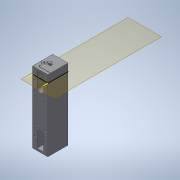
# Autodesk Inventor part: wheel-adapter-front
Saved by Autodesk Inventor 2020 (Build 240168000, 168)
## iProperties
Created: 2020-05-14
Part Number: wheel-adapter-front
Material: Ogólny
Document SubType Name: Modeling
Designer: blep
Density: 1 g/cm^3
Appearance: Domyślna
Author: blep
Autodesk Inventor part; units mm, degrees
ref_plane "YZ Plane" through (0, 0, 0) normal (1, 0, 0) x (0, 1, 0)
ref_plane "XZ Plane" through (0, 0, 0) normal (0, 1, 0) x (-1, 0, 0)
ref_plane "XY Plane" through (0, 0, 0) normal (0, 0, 1) x (1, 0, 0)
ref_plane "Płaszczyzna konstrukcyjna1" through (33, 3, -33.6408) normal (0, 1, 0) x (0, 0, 1)
sketch "Szkic1" plane through (33, 3, -33.6408) normal (0, 1, 0) x (0, 0, 1)
  line L0 (33.6408, -11) -> (70.3592, -11) projected
  line L1 (33.6408, -33) -> (33.6408, -11) projected
  line L2 (33.6408, -11) -> (70.3592, -11)
  line L3 (70.3592, -11) -> (70.3592, -33)
  line L4 (70.3592, -33) -> (33.6408, -33)
  line L5 (33.6408, -33) -> (33.6408, -11)
  constraints: 8 end point, 4 collinear, 2 parallel, 1 horizontal, 1 perpendicular
extrude "Wyciągnięcie proste1" add sketch "Szkic1" against normal blind 3
sketch "Szkic2" plane through (33, 0, -33.6408) normal (0, -1, 0) x (1, 0, 0)
  line L0 (-11, 33.6408) -> (-33, 33.6408)
  line L1 (-33, 33.6408) -> (-33, 39.6408)
  line L2 (-33, 39.6408) -> (-11, 39.6408)
  line L3 (-11, 39.6408) -> (-11, 33.6408)
  line L4 (-33, 33.6408) -> (-11, 33.6408) projected
  line L5 (-11, 33.6408) -> (-11, 70.3592) projected
  line L6 (-33, 70.3592) -> (-33, 33.6408) projected
  dimension "d2" = 6
  constraints: 8 end point, 3 collinear, 2 parallel, 1 horizontal, 1 perpendicular
  measures "d2" distance between parallel lines of L0 L2
extrude "Wyciągnięcie proste2" add sketch "Szkic2" along normal blind 20
sketch "Szkic3" plane through (22, 3, 0) normal (0, 0, -1) x (-1, 0, 0)
  circle A0 centre (18.7, -6) radius 1.25 projected
  circle A1 centre (3.3, -6) radius 1.25 projected
  circle A2 centre (3.3, -20) radius 1.25 projected
  circle A3 centre (18.7, -20) radius 1.25 projected
  circle A4 centre (11, -13) radius 2.125 projected
  circle A5 centre (18.7, -6) radius 1.5
  circle A6 centre (18.7, -20) radius 1.5
  circle A7 centre (3.3, -6) radius 1.5
  circle A8 centre (3.3, -20) radius 1.5
  point P0 (22, -3)
  dimension "d5" = 0.25
  dimension "d6" = 0.25
  dimension "d7" = 0.25
  dimension "d8" = 0.25
  constraints: 4 centre point
  measures "d5" radial gap between concentric circles of A0 A5
  measures "d6" radial gap between concentric circles of A3 A6
  measures "d7" radial gap between concentric circles of A1 A7
  measures "d8" radial gap between concentric circles of A2 A8
extrude "Wyciągnięcie proste3" cut sketch "Szkic3" against normal through all contours A0 | A1 | A2 | A3 | A4 | A5 | A6 | A7 | A8
sketch "Szkic4" plane through (33, 3, -33.6408) normal (0, 1, 0) x (1, 0, 0)
  line L0 (-33, -48.2408) -> (-22, -48.2408) construction
  line L1 (-22, -48.2408) -> (-11, -48.2408) construction
  line L2 (-11, -70.3592) -> (-11, -33.6408) projected
  line L3 (-33, -33.6408) -> (-33, -70.3592) projected
  line L4 (-11, -33.6408) -> (-33, -33.6408) projected
  line L5 (-22, -48.2408) -> (-22, -33.6408) construction
  line L6 (-22, -48.2408) -> (-22, -62.8408) construction
  line L7 (-11, -33.6408) -> (-33, -33.6408)
  line L8 (-33, -33.6408) -> (-33, -62.8408)
  line L9 (-33, -62.8408) -> (-11, -62.8408)
  line L10 (-11, -62.8408) -> (-11, -33.6408)
  point P0 (-11, -62.8408)
  dimension "d11" = 14.6
  constraints: 16 end point, 5 collinear, 3 horizontal, 2 midpoint, 2 parallel, 2 point on line, 2 vertical, 1 perpendicular
  measures "d11" distance from line of L4 L0.end
extrude "Wyciągnięcie proste4" cut sketch "Szkic4" against normal through all keep common part
sketch "Szkic6" plane through (33, 3, -33.6408) normal (0, 1, 0) x (1, 0, 0)
  line L0 (-11, -62.8408) -> (-33, -62.8408) projected
  line L1 (-11, -62.8408) -> (-11, -33.6408) projected
  line L2 (-11, -33.6408) -> (-33, -33.6408) projected
  line L3 (-33, -33.6408) -> (-33, -62.8408) projected
extrude "Wyciągnięcie proste5" add sketch "Szkic6" along normal blind 10.5
hole "Otwór3" at (11, 3, 14.6) direction (0, -1, 0) diameter 4.25 end through all both
sketch "Szkic7" plane through (33, 0, -33.6408) normal (0, -1, 0) x (1, 0, 0)
  circle A0 centre (-22, 48.2408) radius 2.125 projected
  circle A1 centre (-22, 48.2408) radius 4.5
  point P0 (-33, 33.6408)
  dimension "d37" = 9
  constraints: 1 centre point, 1 coincident
  measures "d37" diameter of A1
extrude "Wyciągnięcie proste6" cut sketch "Szkic7" against normal blind 12 contours A0 | A1
sketch "Szkic8" plane through (33, -20, -33.6408) normal (0, -1, 0) x (1, 0, 0)
  line L0 (-33, 33.6408) -> (-11, 33.6408) projected
  line L1 (-11, 33.6408) -> (-11, 39.6408) projected
  line L2 (-11, 39.6408) -> (-33, 39.6408) projected
  line L3 (-33, 39.6408) -> (-33, 33.6408) projected
extrude "Wyciągnięcie proste7" add sketch "Szkic8" along normal blind 18
mirror "Odbij1" about plane through (11, -38, 3) normal (0, -1, 0)
sketch "Szkic9" plane through (0, 0, 6) normal (0, 0, 1) x (1, 0, 0)
  circle A0 centre (11, -66) radius 2.125 projected
  circle A1 centre (18.7, -73) radius 1.5 projected
  circle A2 centre (3.3, -73) radius 1.5 projected
  circle A3 centre (18.7, -59) radius 1.5 projected
  circle A4 centre (3.3, -59) radius 1.5 projected
  circle A5 centre (3.3, -17) radius 1.5 projected
  circle A6 centre (18.7, -17) radius 1.5 projected
  circle A7 centre (3.3, -3) radius 1.5 projected
  circle A8 centre (18.7, -3) radius 1.5 projected
  circle A9 centre (11, -10) radius 2.125 projected
  line L0 (0, 0) -> (22, 0) projected
  line L1 (0, 0) -> (0, -76) projected
  line L2 (0, -76) -> (22, -76) projected
  line L3 (22, 0) -> (22, -76) projected
  circle A10 centre (11, -66) radius 2.125 projected
  circle A11 centre (11, -66) radius 4.5
  circle A12 centre (11, -10) radius 4.5
  point P0 (0, 0)
  dimension "d42" = 9
  dimension "d43" = 9
  constraints: 2 centre point, 2 coincident
  measures "d42" diameter of A11
  measures "d43" diameter of A12
extrude "Wyciągnięcie proste8" add sketch "Szkic9" along normal up to surface (23.2 mm away) contours L0 L3 L2 L1
sketch "Szkic11" plane through (0, 13.5, 29.2) normal (0, 0, 1) x (1, 0, 0)
  line L0 (6.5, -3) -> (15.5, -3)
  line L1 (15.5, -3) -> (15.5, -23.5)
  line L2 (15.5, -23.5) -> (6.5, -23.5)
  line L3 (6.5, -23.5) -> (6.5, -3)
  line L4 (6.5, -79.5) -> (15.5, -79.5)
  line L5 (15.5, -79.5) -> (15.5, -100)
  line L6 (15.5, -100) -> (6.5, -100)
  line L7 (6.5, -100) -> (6.5, -79.5)
  line L8 (0, 0) -> (0, -103) construction
  line L9 (0, 0) -> (6.5, -3) construction
  line L10 (15.5, -3) -> (22, 0) construction
  line L11 (0, 0) -> (22, 0) construction
  line L12 (0, -103) -> (22, -103) construction
  circle A0 centre (11, -23.5) radius 4.5 projected
  circle A1 centre (11, -79.5) radius 4.5 projected
  point P0 (0, -13.5)
  dimension "d48" = 3
  dimension "d51" = 3
  constraints: 20 end point, 4 parallel, 2 collinear, 2 horizontal, 2 horizontal alignment, 2 perpendicular, 1 coincident, 1 equal length, 1 vertical, 2 other
  measures "d48" distance between parallel lines of L11 L0
  measures "d51" distance between parallel lines of L12 L6
extrude "Wyciągnięcie proste9" cut sketch "Szkic11" against normal blind 19.1 contours L0 L1 A0 L3 | A0 L2 | A1 L5 L6 L7 | L4 A1 picked at (12.4564, -23.141) picked at (10.4681, -80.9025)
equation "\"d51\" = d48"
